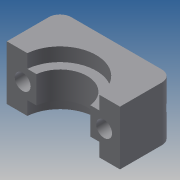
# Autodesk Inventor part: e3d mount
Saved by Autodesk Inventor 2013 (Build 170138000, 138)
## iProperties
Created: 2017-04-01
Part Number: e3d mount
Material: Generic
Document SubType Name: Modeling
Designer: employee
Density: 1 g/cm^3
Author: employee
Autodesk Inventor part; units mm, degrees
ref_plane "YZ Plane" through (0, 0, 0) normal (1, 0, 0) x (0, 1, 0)
ref_plane "XZ Plane" through (0, 0, 0) normal (0, 1, 0) x (-1, 0, 0)
ref_plane "XY Plane" through (0, 0, 0) normal (0, 0, 1) x (1, 0, 0)
sketch "Sketch1" plane through (0, 0, 0) normal (0, 0, 1) x (1, 0, 0)
  line L0 (-12.5, 12.5) -> (12.5, 12.5)
  line L1 (12.5, 12.5) -> (12.5, -12.5)
  line L2 (12.5, -12.5) -> (-12.5, -12.5)
  line L3 (-12.5, -12.5) -> (-12.5, 12.5)
  circle A0 centre (0, 0) radius 8
  point P0 (0, 12.5)
  point P1 (-12.5, 0)
  dimension "d0" = 25
  dimension "d2" = 16
  constraints: 8 end point, 2 midpoint, 2 parallel, 2 perpendicular, 1 centre point, 1 coincident, 1 horizontal, 1 horizontal alignment, 1 vertical alignment
  measures "d0" distance of L2.end L0.start
  measures "d2" diameter of A0
extrude "Extrusion1" add sketch "Sketch1" along normal blind 3
sketch "Sketch2" plane through (0, 0, 3) normal (0, 0, 1) x (1, 0, 0)
  circle A0 centre (0, 0) radius 8 projected
  line L0 (12.5, 12.5) -> (-12.5, 12.5) projected
  line L1 (-12.5, 12.5) -> (-12.5, -12.5) projected
  line L2 (-12.5, -12.5) -> (12.5, -12.5) projected
  line L3 (12.5, -12.5) -> (12.5, 12.5) projected
  circle A1 centre (0, 0) radius 6
  dimension "d5" = 12
  constraints: 1 centre point, 1 coincident
  measures "d5" diameter of A1
extrude "Extrusion2" add sketch "Sketch2" along normal blind 6 contours A0 | L3 L2 L1 L0
sketch "Sketch3" plane through (0, 0, 9) normal (0, 0, 1) x (1, 0, 0)
  line L0 (12.5, 12.5) -> (-12.5, 12.5) projected
  line L1 (-12.5, 12.5) -> (-12.5, -12.5) projected
  line L2 (-12.5, -12.5) -> (12.5, -12.5) projected
  line L3 (12.5, -12.5) -> (12.5, 12.5) projected
  circle A0 centre (0, 0) radius 8 projected
extrude "Extrusion3" add sketch "Sketch3" along normal blind 3
sketch "Sketch4" plane through (0, 0, 12) normal (0, 0, 1) x (1, 0, 0)
  circle A0 centre (0, 0) radius 8 projected
  line L0 (-12.5, 12.5) -> (-12.5, -12.5) projected
  line L1 (-12.5, 0.75) -> (12.5, 0.75)
  line L2 (12.5, 0.75) -> (12.5, -12.5)
  line L3 (12.5, -12.5) -> (-12.5, -12.5)
  line L4 (-12.5, -12.5) -> (-12.5, 0.75)
  dimension "d11" = 0.75
  constraints: 8 end point, 2 parallel, 1 horizontal, 1 perpendicular, 1 point on line
  measures "d11" distance from line of L1 A0.centre
extrude "Extrusion4" cut sketch "Sketch4" against normal through all contours A0 L1 | A0 L1 L2 L3 L0 picked at (-1.088, -1.9346)
sketch "Sketch5" plane through (-12.5, 12.5, 0) normal (0, 1, 0) x (1, 0, 0)
  line L0 (0, 0) -> (0, -12) projected
  line L1 (25, 0) -> (25, -12) projected
  circle A0 centre (3.5, -6) radius 1.75
  circle A1 centre (21.5, -6) radius 1.75
  point P0 (12.5, 0)
  point P1 (25, -6)
  point P2 (0, -6)
  dimension "d14" = 3.5
  dimension "d16" = 3.5
  dimension "d17" = 3.5
  constraints: 2 centre point, 2 horizontal alignment, 2 midpoint, 1 equal radius
  measures "d14" diameter of A0
  measures "d16" distance from line of L0 A0.centre
  measures "d17" distance from line of L1 A1.centre
extrude "Extrusion5" cut sketch "Sketch5" against normal through all
sketch "Sketch6" plane through (-12.5, 12.5, 0) normal (0, 1, 0) x (1, 0, 0)
  circle A0 centre (3.5, -6) radius 1.75 projected
  circle A1 centre (21.5, -6) radius 1.75 projected
  circle A2 centre (3.5, -6) radius 3
  circle A3 centre (21.5, -6) radius 3
  point P0 (12.5, 0)
  dimension "d20" = 6
  dimension "d22" = 6
  constraints: 2 centre point, 2 coincident
  measures "d20" diameter of A2
  measures "d22" diameter of A3
extrude "Extrusion6" cut sketch "Sketch6" against normal blind 3
fillet "Fillet1" radius 2.5 2 edges at (-12.5, 12.5, 6) (12.5, 12.5, 6)
body "Solid1"
